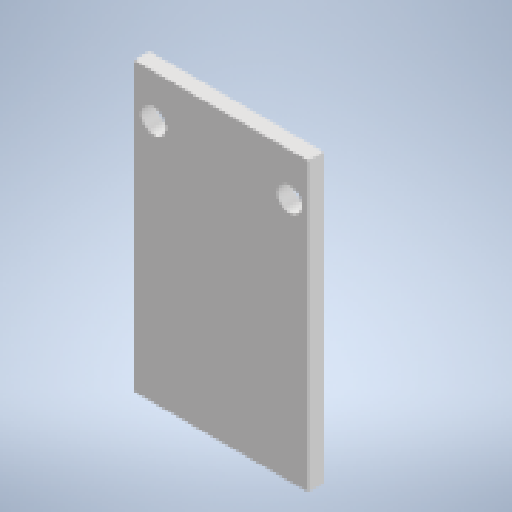
# Autodesk Inventor part: motor_mount
Saved by Autodesk Inventor 2024 (Build 280153000, 153)
## iProperties
Created: 2025-06-20
Part Number: motor_mount
Material: Generic
Document SubType Name: Modeling
Designer: Aidan
Density: 1 g/cm^3
Appearance: Default
Author: Aidan
Autodesk Inventor part; units mm, degrees
ref_plane "YZ Plane" through (0, 0, 0) normal (1, 0, 0) x (0, 1, 0)
ref_plane "XZ Plane" through (0, 0, 0) normal (0, 1, 0) x (-1, 0, 0)
ref_plane "XY Plane" through (0, 0, 0) normal (0, 0, 1) x (1, 0, 0)
sketch "Sketch1" plane through (0, 0, 0) normal (0, 0, 1) x (1, 0, 0)
  circle A0 centre (60.0559, 6.2888) radius 4 projected
  circle A1 centre (60.0559, 6.2888) radius 4
  point P0 (0, 0)
  constraints: 1 centre point, 1 coincident, 1 concentric
extrude "Extrusion1" add sketch "Sketch1" along normal blind 7
sketch "Sketch2" plane through (60.0559, 6.2888, 7) normal (0, 0, 1) x (1, 0, 0)
  line L0 (-11.25, -11.25) -> (11.25, -11.25)
  line L1 (11.25, -11.25) -> (11.25, 25.75)
  line L2 (11.25, 25.75) -> (-11.25, 25.75)
  line L3 (-11.25, 25.75) -> (-11.25, -11.25)
  line L4 (-11.25, -11.25) -> (11.25, 25.75) construction
  line L5 (11.25, -11.25) -> (-11.25, 25.75) construction
  circle A0 centre (0, 0) radius 4 projected
  point P0 (-60.0559, -6.2888)
  point P1 (0, 7.25)
  dimension "d2" = 22.5
  dimension "d3" = 37
  dimension "d4" = 11.25
  dimension "d5" = 11.25
  constraints: 12 end point, 2 midpoint, 2 parallel, 1 horizontal, 1 perpendicular
  measures "d2" distance of L2.end L1.end
  measures "d3" distance of L1.end L0.end
  measures "d4" distance from line of L0 A0.centre
  measures "d5" distance from line of L1 A0.centre
extrude "Extrusion2" add sketch "Sketch2" along normal blind 2 contours L3 L2 L1 L0 | A0
sketch "Sketch3" plane through (60.0559, 6.2888, 9) normal (0, 0, 1) x (1, 0, 0)
  line L0 (11.25, 25.75) -> (-11.25, 25.75) projected
  line L1 (-11.25, 25.75) -> (-11.25, -11.25) projected
  line L2 (11.25, -11.25) -> (11.25, 25.75) projected
  arc A0 (7.3428, 20.8478) -> (8.2491, 21.7255) centre (8.8, 20.25) ccw projected
  arc A1 (-8.1491, 21.7255) -> (-7.2428, 20.8478) centre (-8.7, 20.25) ccw projected
  circle A2 centre (8.8, 20.25) radius 1.575
  circle A3 centre (-8.7, 20.25) radius 1.575
  point P0 (-60.0559, -6.2888)
  point P1 (-7.2428, 20.8478)
  point P2 (-8.1491, 21.7255)
  point P3 (8.2491, 21.7255)
  point P4 (7.3428, 20.8478)
  constraints: 2 centre point, 2 coincident, 2 concentric
extrude "Extrusion3" cut sketch "Sketch3" against normal blind 2
body "Solid1"
